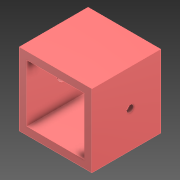
# Autodesk Inventor part: draaideel voor endeffector
Saved by Autodesk Inventor 2020 (Build 240168000, 168)
## iProperties
Created: 2020-05-19
Part Number: draaideel voor endeffector
Material: Generic
Document SubType Name: Modeling
Designer: stefa
Density: 1 g/cm^3
Appearance: Default
Author: stefa
Autodesk Inventor part; units mm, degrees
ref_plane "YZ Plane" through (0, 0, 0) normal (1, 0, 0) x (0, 1, 0)
ref_plane "XZ Plane" through (0, 0, 0) normal (0, 1, 0) x (-1, 0, 0)
ref_plane "XY Plane" through (0, 0, 0) normal (0, 0, 1) x (1, 0, 0)
sketch "Sketch1" plane through (0, 0, 0) normal (0, 0, 1) x (1, 0, 0)
  line L0 (-37.5, -37.5) -> (37.5, -37.5)
  line L1 (37.5, -37.5) -> (37.5, 37.5)
  line L2 (37.5, 37.5) -> (-37.5, 37.5)
  line L3 (-37.5, 37.5) -> (-37.5, -37.5)
  line L4 (-37.5, -37.5) -> (37.5, 37.5) construction
  line L5 (37.5, -37.5) -> (-37.5, 37.5) construction
  line L6 (47.5, 47.5) -> (47.5, -47.5)
  line L7 (47.5, -47.5) -> (-47.5, -47.5)
  line L8 (-47.5, -47.5) -> (-47.5, 47.5)
  line L9 (-47.5, 47.5) -> (47.5, 47.5)
  point P0 (0, 0)
  dimension "d0" = 75
  dimension "d1" = 75
  dimension "d2" = 10
  constraints: 20 end point, 4 parallel, 2 midpoint, 2 perpendicular, 1 horizontal, 3 other
  measures "d0" distance of L2.end L1.end
  measures "d1" distance of L1.end L0.end
  measures "d2" distance between parallel lines of L1 L6
extrude "Extrusion1" add sketch "Sketch1" along normal blind 5 contours L3 L2 L1 L0 | L6 L7 L8 L9
extrude "Extrusion2" add sketch "Sketch1" along normal blind 90
sketch "Sketch5" plane through (-37.5, -37.5, 5) normal (1, 0, 0) x (0, 0, -1)
  circle A0 centre (-35, 37.5) radius 11
  line L0 (5, 85) -> (5, -10) projected
  circle A1 centre (-35, 37.5) radius 4.5
  point P0 (5, 37.5)
  point P1 (5, 37.5)
  dimension "d16" = 22
  dimension "d17" = 40
  dimension "d18" = 9
  constraints: 2 centre point, 1 coincident, 1 horizontal alignment, 1 midpoint
  measures "d16" diameter of A0
  measures "d17" distance from line of A0.centre L0
  measures "d18" diameter of A1
extrude "Extrusion5" cut sketch "Sketch5" against normal blind 7
extrude "Extrusion6" cut sketch "Sketch5" against normal up to surface (10 mm away) contours A1
mirror "Mirror2" about plane through (0, 0, 0) normal (1, 0, 0) of "Extrusion6", "Extrusion5"
body "Solid1"
